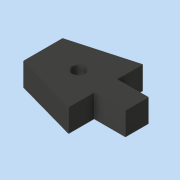
# Autodesk Inventor part: photoTransistor
Saved by Autodesk Inventor 2017 (Build 210142000, 142)
## iProperties
Created: 2016-12-12
Part Number: photoTransistor
Material: ABS Plastic
Document SubType Name: Modeling
Designer: techn
Density: 1.06 g/cm^3
Appearance: Smooth - Black
Author: techn
Autodesk Inventor part; units mm, degrees
ref_plane "YZ Plane" through (0, 0, 0) normal (1, 0, 0) x (0, 1, 0)
ref_plane "XZ Plane" through (0, 0, 0) normal (0, 1, 0) x (-1, 0, 0)
ref_plane "XY Plane" through (0, 0, 0) normal (0, 0, 1) x (1, 0, 0)
sketch "Sketch1" plane through (0, 0, 0) normal (0, 1, 0) x (-1, 0, 0)
  line L0 (0, 0) -> (0, -9.525)
  line L1 (-15.24, 4.2545) -> (-15.24, -13.7795)
  line L2 (0, 0) -> (-15.24, 4.2545)
  line L3 (0, -9.525) -> (-15.24, -13.7795)
  line L4 (-15.24, 4.2545) -> (-19.05, 4.2545)
  line L5 (-19.05, 4.2545) -> (-19.05, 2.9845)
  line L6 (-19.05, 2.9845) -> (-15.24, 2.9845)
  line L7 (-15.24, 2.9845) -> (-15.24, 4.2545)
  line L8 (-15.24, -13.7795) -> (-19.05, -13.7795)
  line L9 (-19.05, -13.7795) -> (-19.05, -12.5095)
  line L10 (-19.05, -12.5095) -> (-15.24, -12.5095)
  line L11 (-15.24, -12.5095) -> (-15.24, -13.7795)
  line L12 (0, 0) -> (0, 3.175)
  line L13 (-15.24, 4.2545) -> (-15.24, 7.4295)
  line L14 (0, -9.525) -> (0, -12.7)
  line L15 (-15.24, -13.7795) -> (-15.24, -16.9545)
  line L16 (-15.24, -16.9545) -> (0, -12.7)
  line L17 (0, 3.175) -> (-15.24, 7.4295)
  line L18 (-15.24, 7.4295) -> (-34.29, 7.4295)
  line L19 (-19.05, 4.2545) -> (-34.29, 4.2545)
  line L20 (-34.29, 4.2545) -> (-34.29, 7.4295)
  line L21 (-15.24, -16.9545) -> (-34.29, -16.9545)
  line L22 (-34.29, -16.9545) -> (-34.29, -13.7795)
  line L23 (-34.29, -13.7795) -> (-19.05, -13.7795)
  line L24 (-34.29, 7.4295) -> (-37.465, 7.4295)
  line L25 (-37.465, 7.4295) -> (-37.465, -17.5895)
  line L26 (-37.465, -17.5895) -> (-34.29, -17.5895)
  line L27 (-34.29, -17.5895) -> (-34.29, 7.4295)
  line L28 (-15.24, -13.7795) -> (-34.29, -13.7795)
  line L29 (-34.29, -13.7795) -> (-34.29, 4.2545)
  line L30 (-34.29, 4.2545) -> (-15.24, 4.2545)
  line L31 (-15.24, 4.2545) -> (-15.24, -13.7795)
  line L32 (-15.24, 4.2545) -> (-34.29, 4.2545)
  line L33 (-34.29, 4.2545) -> (-34.29, 7.4295)
  line L34 (-34.29, 7.4295) -> (-15.24, 7.4295)
  line L35 (-15.24, 7.4295) -> (-15.24, 4.2545)
  line L36 (-15.24, -7.5565) -> (-22.86, -7.5565)
  line L37 (-22.86, -7.5565) -> (-22.86, -1.9685)
  line L38 (-22.86, -1.9685) -> (-15.24, -1.9685)
  line L39 (-15.24, -1.9685) -> (-15.24, -7.5565)
  dimension "d0" = 9.525
  dimension "d1" = 15.24
  dimension "d2" = 18.034
  dimension "d3" = 4.2545
  dimension "d4" = 3.81
  dimension "d5" = 1.27
  dimension "d6" = 3.81
  dimension "d7" = 1.27
  dimension "d8" = 3.175
  dimension "d9" = 3.175
  dimension "d10" = 3.175
  dimension "d11" = 3.175
  dimension "d12" = 19.05
  dimension "d13" = 3.175
  dimension "d30" = 7.62
  dimension "d31" = 5.588
  dimension "d32" = 6.223
  constraints: 80 end point, 13 parallel, 9 perpendicular, 7 horizontal, 6 vertical, 3 point on line
  measures "d0" distance of L0.start L0.end
  measures "d1" distance between parallel lines of L1 L0
  measures "d2" distance of L1.start L1.end
  measures "d3" vertical distance of L1.start L0.start
  measures "d4" distance of L6.end L5.end
  measures "d5" distance of L5.end L4.end
  measures "d6" distance of L9.end L10.end
  measures "d7" distance of L8.end L9.end
  measures "d8" distance of L0.start L12.end
  measures "d9" distance of L1.start L13.end
  measures "d10" distance of L0.end L14.end
  measures "d11" distance of L1.end L15.end
  measures "d12" distance of L13.end L18.end
  measures "d13" distance of L26.end L25.end
  measures "d30" distance of L37.end L38.end
  measures "d31" distance of L36.end L37.end
  measures "d32" distance between parallel lines of L28 L36
extrude "Extrusion6" add sketch "Sketch1" along normal blind 5.588 contours L0 L3 L1 L2 | L1 L36 L37 L38
sketch "Sketch5" plane through (0, 5.588, 0) normal (0, 1, 0) x (1, 0, 0)
  circle A0 centre (8.636, 4.7625) radius 1.5875
  line L0 (0, 9.525) -> (0, 0) projected
  dimension "d35" = 3.175
  dimension "d36" = 8.636
  constraints: 1 centre point
  measures "d35" diameter of A0
  measures "d36" horizontal distance of L0.end A0.centre
extrude "Extrusion7" cut sketch "Sketch5" against normal blind 5.588
equation "\"d3\" = -0.5 * d0 + 0.5 * d2"
equation "\"d32\" = -0.5 * d31 + 0.5 * d2"
body "Solid3"
